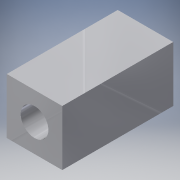
# Autodesk Inventor part: boltholder
Saved by Autodesk Inventor 2016 (Build 200138000, 138)
## iProperties
Created: 2016-01-30
Part Number: boltholder
Material: Aluminum 6061
Document SubType Name: Modeling
Designer: zachary
Density: 2.7 g/cm^3
Appearance: Aluminum - Flat
Mass: 8.88939 g
Surface Area: 20.5627 cm^2
Volume: 3.29237 cm^3
Author: zachary
Autodesk Inventor part; units mm, degrees
ref_plane "YZ Plane" through (0, 0, 0) normal (1, 0, 0) x (0, 1, 0)
ref_plane "XZ Plane" through (0, 0, 0) normal (0, 1, 0) x (-1, 0, 0)
ref_plane "XY Plane" through (0, 0, 0) normal (0, 0, 1) x (1, 0, 0)
sketch "Sketch1" plane through (0, 0, 0) normal (0, 0, 1) x (1, 0, 0)
  line L0 (0, 0) -> (12.7, 0)
  line L1 (12.7, 0) -> (12.7, -12.7)
  line L2 (12.7, -12.7) -> (0, -12.7)
  line L3 (0, -12.7) -> (0, 0)
  circle A0 centre (6.35, -6.35) radius 3.175
  dimension "d0" = 6.35
  dimension "d1" = 12.7
  dimension "d2" = 12.7
  dimension "d3" = 6.35
  dimension "d4" = 6.35
  constraints: 8 end point, 2 parallel, 1 centre point, 1 horizontal, 1 perpendicular
  measures "d0" diameter of A0
  measures "d1" distance of L0.end L1.end
  measures "d2" distance between parallel lines of L3 L1
  measures "d3" distance from line of L1 A0.centre
  measures "d4" distance from line of L2 A0.centre
extrude "Extrusion1" add sketch "Sketch1" along normal blind 25.4
body "Solid1"
